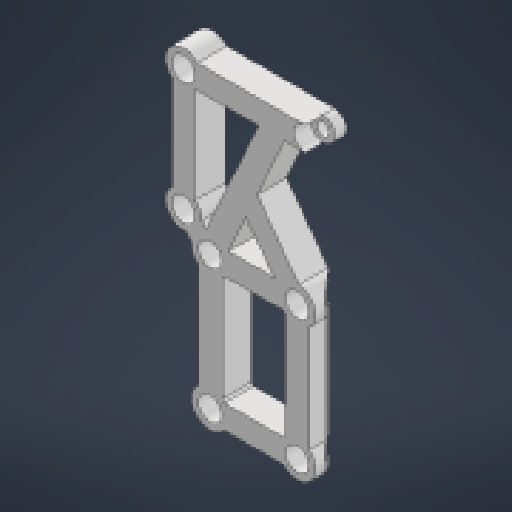
# Autodesk Inventor part: hemera-mount
Saved by Autodesk Inventor 2025 (Build 290162000, 162)
## iProperties
Created: 2024-07-16
Part Number: hemera-mount
Material: Generic
Document SubType Name: Modeling
Designer: Windows 7 was better
Density: 1 g/cm^3
Appearance: Default
Author: Windows 7 was better
Autodesk Inventor part; units mm, degrees
ref_plane "YZ Plane" through (0, 0, 0) normal (1, 0, 0) x (0, 1, 0)
ref_plane "XZ Plane" through (0, 0, 0) normal (0, 1, 0) x (-1, 0, 0)
sketch "Sketch1" plane through (0, 0, 0) normal (0, 0, 1) x (1, 0, 0)
  circle A0 centre (-7, 39.4) radius 1.6
  arc A1 (22.5, 38.8432) -> (22.5, 39.9568) centre (24, 39.4) ccw
  circle A2 centre (-7, 8.4) radius 1.6
  circle A3 centre (-0.2171, 1.8572) radius 1.7
  circle A4 centre (-0.2171, -32.1428) radius 1.7
  circle A5 centre (33.7829, -32.1428) radius 1.7
  circle A6 centre (33.7829, 1.8572) radius 1.7
  line L0 (24, 39.4) -> (-7, 39.4) construction
  line L1 (-7, 39.4) -> (-7, 8.4) construction
  line L2 (-7, 8.4) -> (-0.2171, 1.8572) construction
  line L3 (-0.2171, 1.8572) -> (-0.2171, -32.1428) construction
  line L4 (16.7829, 39.4) -> (-0.2171, 1.8572) construction
  circle A7 centre (-7, 39.4) radius 4.6
  arc A8 (19.6875, 37.7993) -> (19.6875, 41.0007) centre (24, 39.4) ccw
  arc A9 (19.6875, 41.0007) -> (19.6875, 37.7993) centre (24, 39.4) ccw
  circle A10 centre (-7, 8.4) radius 4.6
  circle A11 centre (-0.2171, 1.8572) radius 4.7
  circle A12 centre (-0.2171, -32.1428) radius 4.7
  line L5 (24, 42.4) -> (-7, 42.4)
  line L6 (-7, 42.4) -> (-7, 36.4)
  line L7 (-7, 36.4) -> (24, 36.4)
  line L8 (24, 36.4) -> (24, 42.4)
  line L9 (24, 42.4) -> (-7, 36.4) construction
  line L10 (-7, 42.4) -> (24, 36.4) construction
  line L11 (-10, 39.4) -> (-10, 8.4)
  line L12 (-10, 8.4) -> (-4, 8.4)
  line L13 (-4, 8.4) -> (-4, 39.4)
  line L14 (-4, 39.4) -> (-10, 39.4)
  line L15 (-10, 39.4) -> (-4, 8.4) construction
  line L16 (-10, 8.4) -> (-4, 39.4) construction
  line L17 (-2.95, 3.0947) -> (14.05, 40.6375)
  line L18 (14.05, 40.6375) -> (19.5158, 38.1625)
  line L19 (19.5158, 38.1625) -> (2.5158, 0.6197)
  line L20 (2.5158, 0.6197) -> (-2.95, 3.0947)
  line L21 (-2.95, 3.0947) -> (19.5158, 38.1625) construction
  line L22 (14.05, 40.6375) -> (2.5158, 0.6197) construction
  line L23 (10.0614, 23.0446) -> (6.5044, 18.2126)
  line L24 (-0.2171, -1.1428) -> (-0.2171, 4.8572)
  line L25 (-0.2171, -29.1428) -> (-0.2171, -35.1428)
  line L26 (-3.2171, -32.1428) -> (-3.2171, 1.8572)
  line L27 (-3.2171, 1.8572) -> (2.7829, 1.8572)
  line L28 (2.7829, 1.8572) -> (2.7829, -32.1428)
  line L29 (2.7829, -32.1428) -> (-3.2171, -32.1428)
  line L30 (-3.2171, -32.1428) -> (2.7829, 1.8572) construction
  line L31 (-3.2171, 1.8572) -> (2.7829, -32.1428) construction
  line L32 (-4.8998, 10.5424) -> (1.8656, 4.0164)
  line L33 (1.8656, 4.0164) -> (-2.2999, -0.302)
  line L34 (-2.2999, -0.302) -> (-9.0653, 6.224)
  line L35 (-9.0653, 6.224) -> (-4.8998, 10.5424)
  line L36 (-4.8998, 10.5424) -> (-2.2999, -0.302) construction
  line L37 (1.8656, 4.0164) -> (-9.0653, 6.224) construction
  line L38 (-2.3384, -0.2641) -> (1.9042, 3.9785)
  circle A13 centre (24, 39.4) radius 1.6
  spline S0 degree 3 poles (20.7184, 1.8572) (20.7184, 1.6917) (20.7513, 1.5262) (20.8146, 1.3733) (21.0242, 0.8674) (21.5921, 0.5358) (22.1358, 0.602) (22.578, 0.6558) (22.9807, 0.9617) (23.1511, 1.3733) (23.2145, 1.5262) (23.2474, 1.6916) (23.2474, 1.8572) knots 0 0 0 0 0.071429 0.071429 0.071429 0.307759 0.307759 0.307759 0.500001 0.500001 0.500001 0.57143 0.57143 0.57143 0.57143
  spline S1 degree 3 poles (23.2474, 1.8572) (23.2474, 2.1056) (23.1722, 2.3533) (23.0343, 2.5597) (22.7347, 3.008) (22.1279, 3.2242) (21.6124, 3.0662) (21.4157, 3.006) (21.2342, 2.8968) (21.0887, 2.7514) knots 0 0 0 0 0.25 0.25 0.25 0.792862 0.792862 0.792862 1 1 1 1
  arc A14 (21.0887, 2.7514) -> (20.7184, 1.8572) centre (21.9829, 1.8572) ccw
  circle A15 centre (21.9829, 1.8572) radius 1.6
  circle A16 centre (21.9829, -32.1428) radius 1.6
  circle A17 centre (21.9829, 1.8572) radius 4.6
  circle A18 centre (21.9829, -32.1428) radius 4.6
  line L39 (-0.2171, 1.8572) -> (21.9829, 1.8572) construction
  line L40 (21.9829, 1.8572) -> (21.9829, -32.1428) construction
  line L41 (21.9829, -32.1428) -> (-0.2171, -32.1428) construction
  line L42 (-0.2171, -29.1428) -> (21.9829, -29.1428)
  line L43 (21.9829, -29.1428) -> (21.9829, -35.1428)
  line L44 (21.9829, -35.1428) -> (-0.2171, -35.1428)
  line L45 (-0.2171, -35.1428) -> (-0.2171, -29.1428)
  line L46 (-0.2171, -29.1428) -> (21.9829, -35.1428) construction
  line L47 (21.9829, -29.1428) -> (-0.2171, -35.1428) construction
  line L48 (18.9829, 1.8572) -> (18.9829, -32.1428)
  line L49 (18.9829, -32.1428) -> (24.9829, -32.1428)
  line L50 (24.9829, -32.1428) -> (24.9829, 1.8572)
  line L51 (24.9829, 1.8572) -> (18.9829, 1.8572)
  line L52 (18.9829, 1.8572) -> (24.9829, -32.1428) construction
  line L53 (18.9829, -32.1428) -> (24.9829, 1.8572) construction
  line L54 (-0.2171, 4.8572) -> (21.9829, 4.8572)
  line L55 (21.9829, 4.8572) -> (21.9829, -1.1428)
  line L56 (21.9829, -1.1428) -> (-0.2171, -1.1428)
  line L57 (-0.2171, -1.1428) -> (-0.2171, 4.8572)
  line L58 (-0.2171, 4.8572) -> (21.9829, -1.1428) construction
  line L59 (21.9829, 4.8572) -> (-0.2171, -1.1428) construction
  line L60 (21.9829, 1.8572) -> (8.2829, 20.6286) construction
  line L61 (5.8596, 18.86) -> (19.5596, 0.0886)
  line L62 (19.5596, 0.0886) -> (24.4061, 3.6258)
  line L63 (24.4061, 3.6258) -> (10.7061, 22.3972)
  line L64 (10.7061, 22.3972) -> (5.8596, 18.86)
  line L65 (5.8596, 18.86) -> (24.4061, 3.6258) construction
  line L66 (19.5596, 0.0886) -> (10.7061, 22.3972) construction
  point P0 (0, 0)
  point P1 (8.5, 39.4)
  point P2 (-7, 23.9)
  point P3 (21.0329, 11.2429)
  point P4 (16.7829, 1.8572)
  point P5 (16.7829, -32.1428)
  point P6 (-0.2171, -15.1428)
  point P7 (-3.5998, 5.1202)
  point P8 (-10, 11.8871)
  point P9 (-6.573, 3.8199)
  point P10 (-4.9039, 2.2098)
  point P11 (-3.2171, -1.7608)
  point P12 (-3.2171, -28.5248)
  point P13 (18.7177, 36.4)
  point P14 (20.5129, 36.4)
  point P15 (20.5129, 42.4)
  point P16 (-3.5129, 42.4)
  point P17 (-10, 35.9129)
  point P18 (2.7829, -28.5248)
  point P19 (2.7829, -1.7608)
  point P20 (-4, 36.4)
  point P21 (12.1312, 36.4)
  point P22 (-1.1955, 6.9692)
  point P23 (-0.7383, 6.5282)
  point P24 (-1.4576, 6.3906)
  point P25 (-2.4075, 8.1382)
  point P26 (-4, 11.8871)
  point P27 (16.7829, -15.1428)
  point P28 (10.8829, -32.1428)
  point P29 (21.9829, -15.1428)
  point P30 (10.8829, 1.8572)
  point P31 (-3.5129, 36.4)
  point P32 (-6.9664, 8.4)
  point P33 (-4, 9.6744)
  point P34 (-3.2171, 0.5828)
  point P35 (-0.2171, 1.8572)
  point P36 (-0.2171, 1.8572)
  point P37 (-0.2171, 1.8572)
  point P38 (2.7829, 1.2096)
  point P39 (4.0082, 3.9156)
  point P40 (-4, 35.9129)
  point P41 (18.4958, -35.1428)
  point P42 (24.9829, -28.6557)
  point P43 (24.9829, -1.6299)
  point P44 (18.4958, 4.8572)
  point P45 (4.4346, 4.8572)
  point P46 (3.4009, -1.1428)
  point P47 (18.4958, -1.1428)
  point P48 (18.9829, -1.6299)
  point P49 (18.9829, -28.6557)
  point P50 (18.4958, -29.1428)
  point P51 (3.4009, -29.1428)
  point P52 (3.4009, -35.1428)
  point P53 (-5.8719, 9.5346)
  point P54 (-5.4, 8.4)
  point P55 (-8.6, 39.4)
  point P56 (-7, 37.8)
  point P57 (-1.3973, 0.6337)
  point P58 (-0.2171, 1.8572)
  point P59 (-1.4192, 0.6551)
  point P60 (0.9631, 3.0808)
  point P61 (0.985, 3.0593)
  point P62 (15.1329, 11.2429)
  point P63 (22.3504, 6.4425)
  point P64 (11.7372, 20.9844)
  point P65 (8.8932, 14.7036)
  point P66 (16.0794, 4.8572)
  dimension "d0" = 3
  dimension "d1" = 3
  dimension "d2" = 3
  dimension "d3" = 3
  dimension "d6" = 3
  dimension "d7" = 6
  dimension "d8" = 6
  dimension "d9" = 6
  dimension "d10" = 6
  dimension "d14" = 6
  dimension "d15" = 6
  dimension "d44" = 3.2
  dimension "d45" = 3.2
  dimension "d46" = 3
  dimension "d47" = 3
  dimension "d48" = 6
  dimension "d49" = 6
  dimension "d50" = 6
  dimension "d57" = 6
  constraints: 134 end point, 25 parallel, 24 midpoint, 14 perpendicular, 9 centre point, 4 point on circle, 2 horizontal, 2 point on line, 1 coincident, 4 other
  measures "d0" radial gap between concentric circles of A0 A7
  measures "d1" radial gap between concentric circles of A1 A8
  measures "d2" radial gap between concentric circles of A2 A10
  measures "d6" radial gap between concentric circles of A4 A12
  measures "d7" distance of L6.end L5.end
  measures "d8" distance of L12.end L11.end
  measures "d9" distance of L17.end L18.end
  measures "d10" distance of L23.end L23.start
  measures "d14" distance of L26.end L27.end
  measures "d15" distance of L32.end L33.end
  measures "d44" diameter of A15
  measures "d45" diameter of A16
  measures "d46" radial gap between concentric circles of A15 A17
  measures "d47" radial gap between concentric circles of A16 A18
  measures "d48" distance of L42.end L43.end
  measures "d49" distance of L49.end L48.end
  measures "d50" distance of L54.end L55.end
  measures "d57" distance of L62.end L61.end
extrude "Extrusion1" add sketch "Sketch1" along normal blind 8 contours L14 L13 L7 L6 A0 | A0 L6 L5 A7 L7 L13 L14 | A0 L14 L11 A7 L5 L6 | L6 L7 L13 A7 L11 L14 A0 | L5 A8 A9 L7 L19 L18 L17 A7 | L13 A10 L11 A7 | L5 L8 A1 A13 L7 A8 A9 | A8 L7 L8 A1 L5 | L17 L18 L19 L7 | L7 L19 L63 L64 L61 L54 A11 L32 L17 | L13 L32 L35 A2 L12 L11 A10 | A10 L32 L13 | L11 L12 A2 L35 L34 A10 | L32 A11 L17 | L17 A11 L34 A10 L32 | L32 A10 L34 L35 A2 L12 L13 | L13 L12 A2 L35 L32 | L63 A17 L54 L61 L19 | L19 L61 L64 L63 | L17 L20 A3 L27 L26 L34 A11 | A11 L32 L54 L24 A3 L20 L17 | A11 L54 L32 | L34 L26 A11 | L63 L62 A15 L55 L54 A17 | A17 L50 L51 A15 L62 L63 | L54 L19 A11 | A11 L19 L28 L27 A3 L33 L32 L54 | L32 L33 A3 L24 L54 | L26 L34 L33 A3 L24 L56 L28 A11 | A11 L28 A12 L26 | L26 L27 A3 L38 L34 | L54 L61 A17 L56 A11 L19 | L54 A17 L61 | L54 L55 A15 L51 L48 L61 A17 | A11 L56 L28 L19 | L28 L56 A11 | L26 L29 A4 L25 L44 A12 | A12 L28 L42 L25 A4 L29 L26 | L38 A3 L33 L34 | L61 L48 L56 A17 | L50 A18 L48 A17 | A17 L48 L56 L55 A15 L51 L50 | L28 L56 L24 A3 L20 L19 | L19 L20 A3 L27 L28 | A12 L42 L28 | L44 L25 A4 L29 L28 L42 A12 | A12 L42 A18 L44 | L56 L48 A17 | L61 L62 A15 L55 L56 L48 | L48 L51 A15 L62 L61 | L50 L49 A16 L43 L42 L48 A18 | A18 L44 L43 A16 L49 L50 | L28 L29 A4 L25 L42 | A18 L42 L48 L49 A16 L43 L44 | L48 L42 A18 | L42 L43 A16 L49 L48
ref_plane "Work Plane1" through (25.5, 25.5, 3.75) normal (-0.7808688, 0, 0.624695) x (0, -1, 0)
sketch "Sketch2" plane through (25.5, 25.5, 3.75) normal (-0.7808688, 0, 0.624695) x (0, -1, 0)
  line L0 (64.6935, -4.8599) -> (10.3184, -4.8599)
  line L1 (10.3184, -4.8599) -> (10.3184, 6.1401)
  line L2 (10.3184, 6.1401) -> (64.6935, 6.1401)
  line L3 (64.6935, 6.1401) -> (64.6935, -4.8599)
  point P0 (25.5, -18.858)
  dimension "d19" = 11
  constraints: 8 end point, 2 parallel, 1 horizontal, 1 perpendicular
  measures "d19" distance of L0.end L1.end
extrude "Extrusion2" cut sketch "Sketch2" against normal blind 22.75
sketch "Sketch6" plane through (0, 0, 8) normal (0, 0, 1) x (1, 0, 0)
  arc A0 (-5.8719, 9.5346) -> (-5.8719, 9.5346) centre (-7, 8.4) ccw projected
  arc A1 (-8.6, 39.4) -> (-8.6, 39.4) centre (-7, 39.4) ccw projected
  circle A2 centre (24, 39.4) radius 1.6 projected
  circle A3 centre (-7, 39.4) radius 3
  circle A4 centre (-7, 8.4) radius 3
  circle A5 centre (24, 39.4) radius 3
  point P0 (0, 0)
  dimension "d35" = 6
  dimension "d36" = 6
  dimension "d37" = 6
  constraints: 3 centre point, 3 coincident
  measures "d35" diameter of A3
  measures "d36" diameter of A4
  measures "d37" diameter of A5
extrude "Extrusion6" cut sketch "Sketch6" against normal blind 3.5 contours A0 | A1 | A2 | A3 | A4 | A5
sketch "Sketch7" plane through (0, 0, 8) normal (0, 0, 1) x (1, 0, 0)
  circle A0 centre (24, 39.4) radius 1.6 projected
  circle A1 centre (24, 39.4) radius 3
  arc A2 (20.5129, 36.4) -> (20.5129, 42.4) centre (24, 39.4) ccw projected
  circle A3 centre (24, 39.4) radius 4.6
  line L0 (24, 36.4) -> (20.5129, 36.4)
  line L1 (24, 42.4) -> (20.5129, 42.4)
  point P0 (0, 0)
  dimension "d41" = 6
  constraints: 4 end point, 2 centre point, 2 coincident, 2 point on circle, 1 horizontal, 1 tangent
  measures "d41" diameter of A1
extrude "Extrusion7" cut sketch "Sketch7" against normal blind 9.5 contours A1 L1 A2 L0
sketch "Sketch8" plane through (0, 0, 0) normal (0, 0, -1) x (-1, 0, 0)
  arc A0 (-22.5, 0.3431) -> (-22.5, 3.3713) centre (-21.9829, 1.8572) ccw projected
  circle A1 centre (0.2171, 1.8572) radius 1.7 projected
  circle A2 centre (0.2171, -32.1428) radius 1.7 projected
  arc A3 (-22.5, -33.6569) -> (-22.5, -30.6287) centre (-21.9829, -32.1428) ccw projected
  arc A4 (-22.5, -30.6287) -> (-22.5, -33.6569) centre (-21.9829, -32.1428) ccw projected
  circle A5 centre (-21.9829, -32.1428) radius 3
  circle A6 centre (0.2171, -32.1428) radius 3
  circle A7 centre (0.2171, 1.8572) radius 3
  circle A8 centre (-21.9829, 1.8572) radius 3
  point P0 (0, 0)
  dimension "d51" = 6
  dimension "d52" = 6
  dimension "d53" = 6
  dimension "d54" = 6
  constraints: 4 centre point, 4 coincident
  measures "d51" diameter of A5
  measures "d52" diameter of A6
  measures "d53" diameter of A7
  measures "d54" diameter of A8
extrude "Extrusion8" cut sketch "Sketch8" against normal blind 3 contours A2 | A4 A3 | A5 | A6 | A7 | A8
body "Solid1"
